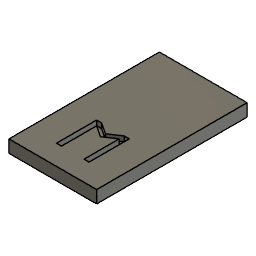
Tapa_M (Autodesk Fusion 360 design; units mm, degrees)
part number: 2025-11-07-13-48-39-675
Autodesk Fusion 360 part; units mm, degrees
sketch "Boceto1" plane through (0, 0, 0) normal (0, 1, 0) x (1, 0, 0)
  line L0 (-50, 50) -> (-50, -10)
  line L1 (-50, 50) -> (-15, 50)
  line L2 (-15, 50) -> (-15, -10)
  line L3 (-15, -10) -> (-50, -10)
  dimension "d1" = 60
  dimension "d2" = 35
  constraint vertical L0
  constraint perpendicular L0 L1
  constraint perpendicular L1 L2
  constraint perpendicular L0 L3
  measures "d1" distance of L0.start L0.end
  measures "d2" distance of L0.start L1.end
extrude "Extruir1" add sketch "Boceto1" along normal blind 3
sketch "Boceto2" plane through (0, 0, 0) normal (0, -1, 0) x (1, 0, 0)
  line L0 (-50, 10) -> (-50, -50)
  line L1 (-50, -50) -> (-15, -50)
  line L2 (-15, -50) -> (-15, 10)
  line L3 (-15, 10) -> (-50, 10)
  line L4 (-35.5, -40) -> (-34.4961, -23.8757)
  line L5 (-29.5, -40) -> (-30.5039, -23.8757)
  arc A0 (-30.5039, -23.8757) -> (-34.4961, -23.8757) centre (-32.5, -24) ccw
  arc A1 (-35.5, -40) -> (-29.5, -40) centre (-32.5, -40) ccw
  arc A2 (-35.5, -40) -> (-29.5, -40) centre (-32.5, -40) ccw
  constraint coincident A1.centre A2.centre
extrude "Extruir2" add 1 faces at (-38.3333, 3, -30) along direction (0, 1, 0) blind 2
extrude "Extruir3" cut sketch "Boceto2" against normal blind 2 contours L4 L5 A0 A1 A2
sketch "Boceto3" plane through (0, 5, 0) normal (0, 1, 0) x (-1, 0, 0)
  line L0 (50, -50) -> (50, 10)
  line L1 (50, 10) -> (15, 10)
  line L2 (15, 10) -> (15, -50)
  line L3 (15, -50) -> (50, -50)
  line L4 (39, -12) -> (39, 2)
  line L5 (39, 2) -> (37, 2)
  line L6 (37, 2) -> (37, -12)
  line L7 (50, 10) -> (32.5, 10)
  line L8 (32.5, -9) -> (37, -12)
  line L9 (28, 2) -> (26, 2)
  line L10 (26, 2) -> (26, -12)
  line L11 (28, 2) -> (28, -12)
  line L12 (28, -12) -> (32.5, -9)
  line L13 (39, -12) -> (39, -14)
  line L14 (39, -14) -> (37, -14)
  line L15 (37, -14) -> (32.5, -11)
  line L16 (32.5, -11) -> (28, -14)
  line L17 (28, -14) -> (26, -14)
  line L18 (26, -14) -> (26, -12)
  constraint parallel L0 L4
  constraint perpendicular L4 L5
  constraint perpendicular L5 L6
  constraint coincident L0.end L1.start
  constraint midpoint L1 L7.end
  constraint perpendicular L9 L10
  constraint perpendicular L9 L11
  constraint parallel L4 L13
  constraint perpendicular L13 L14
  constraint parallel L8 L15
  constraint parallel L12 L16
  constraint parallel L14 L17
  constraint perpendicular L17 L18
extrude "Extruir4" cut sketch "Boceto3" against normal blind 2 contours L4 L5 L6 L8 L9 L10 L11 L12 L13 L14 L15 L16 L17 L18
